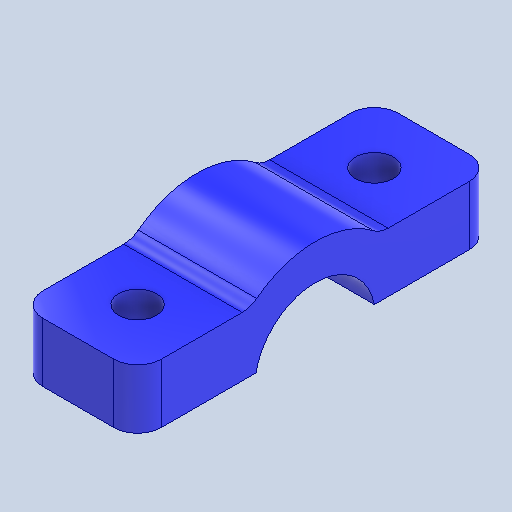
# Autodesk Inventor part: belt_liner_v5_3DP_P-2
Saved by Autodesk Inventor 2025.2 (Build 292293000, 293)
## iProperties
Created: 2025-03-19
Part Number: belt_liner_v5_3DP_P-2
Material: ABS プラスチック
Document SubType Name: Modeling
Designer: haruy
Density: 1.06 g/cm^3
Appearance: 青 - 壁塗料 - 光沢
Author: haruy
Autodesk Inventor part; units mm, degrees
ref_plane "YZ Plane" through (0, 0, 0) normal (1, 0, 0) x (0, 1, 0)
ref_plane "XZ Plane" through (0, 0, 0) normal (0, 1, 0) x (-1, 0, 0)
ref_plane "XY Plane" through (0, 0, 0) normal (0, 0, 1) x (1, 0, 0)
sketch "スケッチ1" plane through (0, 0, 0) normal (1, 0, 0) x (0, 1, 0)
  circle A0 centre (0, 0) radius 5.1
  line L0 (1, 15) -> (6, 15)
  line L1 (6, 15) -> (6, -15)
  line L2 (6, -15) -> (1, -15)
  line L3 (1, -15) -> (1, 15)
  circle A1 centre (0, 0) radius 8.1
  point P0 (1, 5.001)
  point P1 (1, -5.001)
  point P2 (6, -5.4415)
  point P3 (6, 5.4415)
  dimension "d0" = 10.2
  dimension "d1" = 1
  dimension "d2" = 30
  dimension "d3" = 15
  dimension "d4" = 5
  dimension "d5" = 3
  constraints: 8 end point, 2 centre point, 2 parallel, 1 coincident, 1 horizontal, 1 perpendicular
  measures "d0" diameter of A0
  measures "d1" distance from line of L3 point (0, 0)
  measures "d2" distance between parallel lines of L2 L0
  measures "d3" distance from line of L0 point (0, 0)
  measures "d4" distance between parallel lines of L3 L1
  measures "d5" radial gap between concentric circles of A0 A1
extrude "押し出し1" add sketch "スケッチ1" against normal blind 10 contours A0 L3 A1 L1 | L3 L0 L1 A1 | A1 L1 L2 L3 | A1 L1
sketch "スケッチ2" plane through (0, 6, 15) normal (0, 1, 0) x (1, 0, 0)
  line L0 (0, 9.5585) -> (0, 0) projected
  line L1 (0, 0) -> (-10, 0) projected
  line L2 (0, 30) -> (0, 20.4415) projected
  line L3 (0, 30) -> (-10, 30) projected
  point P0 (0, 15)
  point P1 (-5, 5)
  point P2 (-5, 25)
  dimension "d8" = 5
  dimension "d9" = 5
  dimension "d10" = 5
  dimension "d11" = 5
  measures "d8" distance from line of point (-5, 5) L0
  measures "d9" distance from line of point (-5, 5) L1
  measures "d10" distance from line of point (-5, 25) L2
  measures "d11" distance from line of L3 point (-5, 25)
hole "穴1" at (-5, 6, 10) at (-5, 6, -10) direction (0, -1, 0) diameter 3.2 end through all
fillet "フィレット1" radius 2 6 edges at (0, 3.5, 15) (-10, 3.5, 15) (-5, 6, 5.4415) (-5, 6, -5.4415) (0, 3.5, -15) (-10, 3.5, -15)
